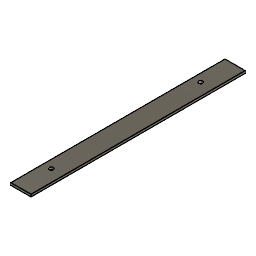
25x265 Banding (Autodesk Fusion 360 design; units mm, degrees)
part number: 2026-06-02-18-18-49-189
Autodesk Fusion 360 part; units mm, degrees
sketch "Sketch1" plane through (0, 0, 0) normal (0, 0, 1) x (1, 0, 0)
  line L0 (12.5, -132.5) -> (-12.5, -132.5)
  line L1 (-12.5, -132.5) -> (-12.5, 132.5)
  line L2 (-12.5, 132.5) -> (12.5, 132.5)
  line L3 (12.5, 132.5) -> (12.5, -132.5)
  line L4 (12.5, -132.5) -> (-12.5, 132.5) construction
  line L5 (-12.5, -132.5) -> (12.5, 132.5) construction
  dimension "d1" = 25
  dimension "d2" = 265
  constraint horizontal L0
  constraint perpendicular L0 L1
  constraint parallel L0 L2
  constraint parallel L1 L3
  constraint coincident L4 origin
  constraint coincident L5 origin
  measures "d1" distance of L1.end L2.end
  measures "d2" distance of L0.end L1.end
extrude "Extrude1" add sketch "Sketch1" along normal blind 3
hole "Hole1" at (-2.5, 92.5, 3) direction (0, 0, -1) diameter 5 depth 65 tip angle 118
hole "Hole2" at (-2.5, -92.5, 3) direction (0, 0, -1) diameter 5 depth 65 tip angle 118
